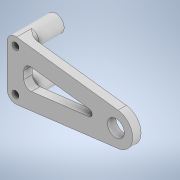
# Autodesk Inventor part: sensor_holder_1
Saved by Autodesk Inventor 2020 (Build 240168000, 168)
## iProperties
Created: 2019-10-15
Part Number: sensor_holder_1
Material: Generic
Document SubType Name: Modeling
Designer: psrob
Density: 1 g/cm^3
Appearance: Default
Author: psrob
Autodesk Inventor part; units mm, degrees
ref_plane "YZ Plane" through (0, 0, 0) normal (1, 0, 0) x (0, 1, 0)
ref_plane "XZ Plane" through (0, 0, 0) normal (0, 1, 0) x (-1, 0, 0)
ref_plane "XY Plane" through (0, 0, 0) normal (0, 0, 1) x (1, 0, 0)
sketch "Sketch1" plane through (0, 0, 0) normal (0, 0, 1) x (1, 0, 0)
  circle A0 centre (6, -12.5) radius 2 projected
  circle A1 centre (6, 12.5) radius 2 projected
  circle A2 centre (-10, -12.5) radius 2 projected
  circle A3 centre (-10, 12.5) radius 2 projected
  circle A4 centre (18, 0) radius 2.1 projected
  circle A5 centre (28, 0) radius 2.1 projected
  circle A6 centre (38, 0) radius 2.1 projected
  circle A7 centre (50, 0) radius 6.5 projected
  circle A8 centre (0, -12.5) radius 1.5 projected
  circle A9 centre (0, 12.5) radius 1.5 projected
  circle A10 centre (0, 0) radius 9 projected
  line L0 (-6.5245, 22) -> (6.5245, 22) projected
  arc A11 (-8.1489, 20.9725) -> (-6.5245, 22) centre (-9.9598, 25.633) ccw projected
  arc A12 (-8.1489, 20.9725) -> (-20.9725, 8.1489) centre (0, 0) ccw projected
  arc A13 (-22, 6.5245) -> (-20.9725, 8.1489) centre (-25.633, 9.9598) ccw projected
  line L1 (-22, -6.5245) -> (-22, 6.5245) projected
  arc A14 (-20.9725, -8.1489) -> (-22, -6.5245) centre (-25.633, -9.9598) ccw projected
  arc A15 (-20.9725, -8.1489) -> (-8.1489, -20.9725) centre (0, 0) ccw projected
  arc A16 (-6.5245, -22) -> (-8.1489, -20.9725) centre (-9.9598, -25.633) ccw projected
  line L2 (6.5245, -22) -> (-6.5245, -22) projected
  arc A17 (8.1489, -20.9725) -> (6.5245, -22) centre (9.9598, -25.633) ccw projected
  arc A18 (8.1489, -20.9725) -> (19.9602, -10.3846) centre (0, 0) ccw projected
  arc A19 (28.8314, -5) -> (19.9602, -10.3846) centre (28.8314, -15) ccw projected
  line L3 (28.8314, -5) -> (33.4169, -5) projected
  arc A20 (44.4723, -8.3333) -> (33.4169, -5) centre (33.4169, -25) ccw projected
  arc A21 (44.4723, -8.3333) -> (44.4723, 8.3333) centre (50, 0) ccw projected
  arc A22 (33.4169, 5) -> (44.4723, 8.3333) centre (33.4169, 25) ccw projected
  line L4 (33.4169, 5) -> (28.8314, 5) projected
  arc A23 (19.9602, 10.3846) -> (28.8314, 5) centre (28.8314, 15) ccw projected
  arc A24 (19.9602, 10.3846) -> (8.1489, 20.9725) centre (0, 0) ccw projected
  arc A25 (6.5245, 22) -> (8.1489, 20.9725) centre (9.9598, 25.633) ccw projected
  circle A26 centre (-10, -12.5) radius 5
  circle A27 centre (-10, 12.5) radius 5
  dimension "d0" = 10
  dimension "d1" = 10
  constraints: 2 centre point, 2 coincident
  measures "d0" diameter of A26
  measures "d1" diameter of A27
extrude "Extrusion1" add sketch "Sketch1" along normal blind 20 contours A26 | A27
sketch "Sketch2" plane through (-10, -12.5, 20) normal (0, 0, 1) x (1, 0, 0)
  circle A0 centre (60, 12.5) radius 2.5 projected
  circle A1 centre (60, 12.5) radius 10
  circle A2 centre (60, 12.5) radius 5
  circle A3 centre (0, 0) radius 5 projected
  circle A4 centre (0, 0) radius 2 projected
  circle A5 centre (0, 25) radius 5 projected
  circle A6 centre (0, 25) radius 2 projected
  line L0 (60, 12.5) -> (-0.617, 4.9618)
  circle A7 centre (0, 0) radius 5 projected
  line L1 (60, 12.5) -> (-0.617, 20.0382)
  line L2 (0, 25) -> (-0.617, 20.0382)
  line L3 (0, 0) -> (-0.617, 4.9618)
  line L4 (61.2341, 2.5764) -> (0.617, -4.9618)
  line L5 (0, 0) -> (0.617, -4.9618)
  line L6 (60, 12.5) -> (61.2341, 2.5764)
  line L7 (61.2341, 22.4236) -> (0.617, 29.9618)
  circle A8 centre (0, 25) radius 5 projected
  line L8 (0, 25) -> (0.617, 29.9618)
  line L9 (61.2341, 22.4236) -> (60, 12.5)
  point P0 (10, 12.5)
  point P1 (50.0764, 13.7341)
  point P2 (50.0764, 11.2659)
  point P3 (-0.617, 4.9618)
  point P4 (0.617, -4.9618)
  point P5 (0.617, 29.9618)
  dimension "d4" = 20
  dimension "d5" = 10
  constraints: 20 end point, 6 perpendicular, 5 point on circle, 3 coincident, 2 centre point, 2 other
  measures "d4" diameter of A1
  measures "d5" diameter of A2
extrude "Extrusion2" add sketch "Sketch2" along normal blind 4 contours L9 A1 L6 A2 | A2 L1 A1 L9 | L6 A1 L0 A2 | A2 L0 A1 L1 | A1 L1 A5 L7 | L4 A3 L0 A1
sketch "Sketch3" plane through (0, 0, 20) normal (0, 0, 1) x (1, 0, 0)
  arc A0 (-10.617, 7.5382) -> (-9.383, 17.4618) centre (-10, 12.5) ccw projected
  arc A1 (-9.383, 17.4618) -> (-10.617, 7.5382) centre (-10, 12.5) ccw projected
  circle A2 centre (-10, 12.5) radius 2 projected
  arc A3 (-9.383, -17.4618) -> (-10.617, -7.5382) centre (-10, -12.5) ccw projected
  arc A4 (-10.617, -7.5382) -> (-9.383, -17.4618) centre (-10, -12.5) ccw projected
  circle A5 centre (-10, -12.5) radius 2 projected
  line L0 (-10, 12.5) -> (-15, 12.5)
  circle A6 centre (-10, 12.5) radius 5 projected
  line L1 (-10, -12.5) -> (-15, -12.5)
  line L2 (-15, -12.5) -> (-15, 12.5)
  line L3 (-10, 12.5) -> (-5, 12.5)
  line L4 (-5, 12.5) -> (-5, -12.5)
  line L5 (-10, -12.5) -> (-5, -12.5)
  point P0 (0, 0)
  constraints: 12 end point, 4 point on circle, 3 perpendicular, 2 horizontal, 1 point on line
extrude "Extrusion3" add sketch "Sketch3" along normal blind 4 contours A1 L0 A2 L3 A0 | A0 L4 A3 A4 L2 A1 | L3 A2 L0 A1 A0 | L5 A5 L1 A4 A3 | A3 A4 L1 A5 L5
thicken "Thicken1" operation add thickness 1 both sides no extend neighbours yes toward (0, 0, -1) faces at (28.58, -8.659, 20)
thicken "Thicken2" operation add thickness 3 both sides no extend neighbours yes toward (-0.9953736, 0.0960805, 0) faces at (40.0463, 0.9608, 22.3333)
fillet "Fillet1" radius 4 2 edges at (-5, 6.8397, 21.5) (-5, -6.8397, 21.5)
fillet "Fillet2" radius 4 4 edges at (-10, 7.5, 19) (-6.2527, 15.8102, 19) (-6.2527, -15.8102, 19) (-10, -7.5, 19)
fillet "Fillet3" radius 2 2 edges at (37.0994, 1.6043, 21.5) (37.0994, -1.6043, 21.5)
body "Solid1"
